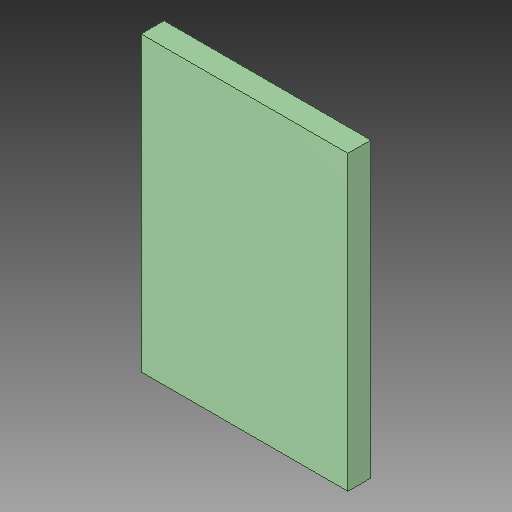
# Autodesk Inventor part: REG-AMS1117-3P-3_3V
Saved by Autodesk Inventor 2019 (Build 230136000, 136)
## iProperties
Created: 2019-10-02
Part Number: REG-AMS1117-3P-3_3V
Material: Generic
Document SubType Name: Modeling
Designer: rybit
Density: 1 g/cm^3
Appearance: REG-AMS1117-3P, REG-AMS1117-3P-3_3V
Author: rybit
Autodesk Inventor part; units mm, degrees
ref_plane "YZ Plane" through (0, 0, 0) normal (1, 0, 0) x (0, 1, 0)
ref_plane "XZ Plane" through (0, 0, 0) normal (0, 1, 0) x (-1, 0, 0)
ref_plane "XY Plane" through (0, 0, 0) normal (0, 0, 1) x (1, 0, 0)
sketch "REG-AMS1117-3P, REG-AMS1117-3P-3_3V_25" plane through (0, 0, 0) normal (0, 0, 1) x (1, 0, 0)
  line L0 (-4.5085, 6.35) -> (4.5085, 6.35)
  line L1 (4.5085, 6.35) -> (4.5085, -6.4135)
  line L2 (4.5085, -6.4135) -> (-4.5085, -6.4135)
  line L3 (-4.5085, -6.4135) -> (-4.5085, 6.35)
  constraints: 8 end point
extrude "Extrusion1" add sketch "REG-AMS1117-3P, REG-AMS1117-3P-3_3V_25" along normal blind 1
body "Solid1"
